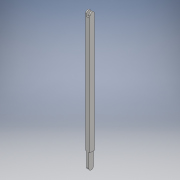
# Autodesk Inventor part: 滑桿
Saved by Autodesk Inventor 2017 (Build 210142000, 142)
## iProperties
Part Number: 滑桿
Material: 一般
Document SubType Name: Modeling
Designer: Brian
Density: 1 g/cm^3
Appearance: 預設
Author: Brian
Autodesk Inventor part; units mm, degrees
ref_plane "YZ Plane" through (0, 0, 0) normal (1, 0, 0) x (0, 1, 0)
ref_plane "XZ Plane" through (0, 0, 0) normal (0, 1, 0) x (-1, 0, 0)
ref_plane "XY Plane" through (0, 0, 0) normal (0, 0, 1) x (1, 0, 0)
sketch "草圖3" plane through (0, 0, 0) normal (0, 0, 1) x (1, 0, 0)
  line L0 (-5, -5) -> (5, -5)
  line L1 (5, -5) -> (5, 5)
  line L2 (5, 5) -> (-5, 5)
  line L3 (-5, 5) -> (-5, -5)
  line L4 (-5, -5) -> (5, 5) construction
  line L5 (5, -5) -> (-5, 5) construction
  point P0 (0, 0)
  dimension "d6" = 10
  dimension "d7" = 10
  constraints: 12 end point, 2 midpoint, 2 parallel, 1 horizontal, 1 perpendicular
  measures "d6" distance of L1.end L2.end
  measures "d7" distance of L2.end L0.start
extrude "擠出3" add sketch "草圖3" along normal blind 300
sketch "草圖4" plane through (0, 0, 300) normal (0, 0, 1) x (1, 0, 0)
  line L0 (-2.5, 10.267) -> (2.5, 10.267)
  line L1 (2.5, 10.267) -> (2.5, -8.2963)
  line L2 (2.5, -8.2963) -> (-2.5, -8.2963)
  line L3 (-2.5, -8.2963) -> (-2.5, 10.267)
  point P0 (0, 0)
  dimension "d10" = 5
  dimension "d11" = 2.5
  constraints: 8 end point, 2 parallel, 1 horizontal, 1 perpendicular
  measures "d10" distance of L0.start L0.end
  measures "d11" distance from line of point (0, 0) L3
extrude "擠出4" cut sketch "草圖4" against normal blind 10
fillet "圓角1" radius 5 4 edges at (3.75, 5, 300) (-3.75, 5, 300) (-3.75, -5, 300) (3.75, -5, 300)
sketch "草圖5" plane through (-5, 5, 0) normal (0, 1, 0) x (1, 0, 0)
  line L0 (-3.8265, -36.4286) -> (2.5, -36.4286)
  line L1 (2.5, -36.4286) -> (2.5, 10.3061)
  line L2 (2.5, 10.3061) -> (-3.8265, 10.3061)
  line L3 (-3.8265, 10.3061) -> (-3.8265, -36.4286)
  line L4 (7.5, -36.4286) -> (18.7245, -36.4286)
  line L5 (18.7245, -36.4286) -> (18.7245, 20.7143)
  line L6 (18.7245, 20.7143) -> (7.5, 20.7143)
  line L7 (7.5, 20.7143) -> (7.5, -36.4286)
  point P0 (5, 0)
  dimension "d15" = 5
  dimension "d16" = 2.5
  constraints: 16 end point, 4 parallel, 2 horizontal, 2 perpendicular, 1 point on line
  measures "d15" distance between parallel lines of L1 L7
  measures "d16" distance from line of point (5, 0) L7
extrude "擠出5" cut sketch "草圖5" against normal blind 15
fillet "圓角2" radius 5 2 edges at (0, 5, 0) (0, -5, 0)
